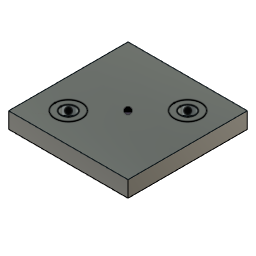
TPU Feet (Autodesk Fusion 360 design; units mm, degrees)
Autodesk Fusion 360 part; units mm, degrees
sketch "Sketch1" plane through (0, 0, 0) normal (0, 0, 1) x (1, 0, 0)
  line L0 (20, -20) -> (-20, -20)
  line L1 (-20, -20) -> (-20, 20)
  line L2 (-20, 20) -> (20, 20)
  line L3 (20, 20) -> (20, -20)
  line L4 (20, -20) -> (-20, 20) construction
  line L5 (-20, -20) -> (20, 20) construction
  dimension "d1" = 40
  dimension "d2" = 40
  constraint horizontal L0
  constraint perpendicular L0 L1
  constraint parallel L0 L2
  constraint parallel L1 L3
  constraint coincident L4 origin
  constraint coincident L5 origin
  measures "d1" distance of L1.end L2.end
  measures "d2" distance of L0.end L1.end
extrude "Extrude1" add sketch "Sketch1" along normal blind 5
chamfer "Chamfer1" distance 8 angle 30 4 edges at (20, 0, 0) (0, -20, 0) (-20, 0, 0) (0, 20, 0) measured on face at (6.6667, -6.6667, 0) measured on face at (6.6667, -6.6667, 0) measured on face at (6.6667, -6.6667, 0) measured on face at (6.6667, -6.6667, 0)
extrude "Extrude2" add 1 faces at (6.6667, -6.6667, 5) along direction (0, 0, 1) blind 5
sketch "Sketch2" plane through (0, 0, 10) normal (0, 0, 1) x (-1, 0, 0)
  line L0 (-20, -20) -> (20, -20)
  line L1 (20, -20) -> (20, 20)
  line L2 (20, 20) -> (-20, 20)
  line L3 (-20, 20) -> (-20, -20)
  circle A0 centre (10, 10) radius 2.5
  circle A1 centre (-10, -10) radius 2.5
  circle A2 centre (10, 10) radius 4.5
  circle A3 centre (-10, -10) radius 4.5
  dimension "d11" = 5
  dimension "d12" = 5
  dimension "d15" = 9
  dimension "d16" = 9
  dimension "d20" = 10
  dimension "d21" = 10
  dimension "d22" = 10
  dimension "d23" = 10
  constraint concentric A0 A2
  constraint concentric A1 A3
  measures "d11" diameter of A0
  measures "d12" diameter of A1
  measures "d15" diameter of A2
  measures "d16" diameter of A3
  measures "d20" distance of L1 A0.centre
  measures "d21" distance of L2 A0.centre
  measures "d22" distance of L0 A1.centre
  measures "d23" distance of L3 A1.centre
extrude "Extrude4" cut sketch "Sketch2" along normal blind 7 from surface at -10 contours A2 | A3
extrude "Extrude3" cut sketch "Sketch2" against normal up to surface (10 mm away) contours A0 | A1
